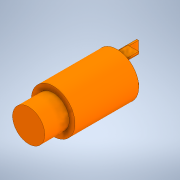
# Autodesk Inventor part: StereoBuchseEinbau
Saved by Autodesk Inventor 2020 (Build 240168000, 168)
## iProperties
Created: 2020-02-17
Part Number: StereoBuchseEinbau
Material: Generic
Document SubType Name: Modeling
Designer: Timo
Density: 1 g/cm^3
Appearance: Default
Author: Timo
Autodesk Inventor part; units mm, degrees
ref_plane "YZ Plane" through (0, 0, 0) normal (1, 0, 0) x (0, 1, 0)
ref_plane "XZ Plane" through (0, 0, 0) normal (0, 1, 0) x (-1, 0, 0)
ref_plane "XY Plane" through (0, 0, 0) normal (0, 0, 1) x (1, 0, 0)
sketch "Sketch1" plane through (0, 0, 0) normal (0, 0, 1) x (1, 0, 0)
  circle A0 centre (0, 0) radius 2.95
  dimension "d0" = 5.9
  constraints: 1 centre point, 1 coincident
  measures "d0" diameter of A0
extrude "Extrusion1" add sketch "Sketch1" along normal blind 4.5
sketch "Sketch2" plane through (0, 0, 0) normal (0, 0, -1) x (-1, 0, 0)
  circle A0 centre (0, 0) radius 4
  dimension "d3" = 8
  constraints: 1 centre point, 1 coincident
  measures "d3" diameter of A0
extrude "Extrusion2" add sketch "Sketch2" along normal blind 11.7
sketch "Sketch3" plane through (0, 0, -11.7) normal (0, 0, -1) x (-1, 0, 0)
  line L0 (2.665, 1.1) -> (2.335, 1.1)
  line L1 (2.335, 1.1) -> (2.335, -1.1)
  line L2 (2.335, -1.1) -> (2.665, -1.1)
  line L3 (2.665, -1.1) -> (2.665, 1.1)
  line L4 (2.5, 1.1) -> (2.5, -1.1) construction
  line L5 (5.6, 0) -> (-5.6, 0) construction
  point P0 (0, 0)
  point P1 (2.5, 0)
  dimension "d6" = 0.33
  dimension "d7" = 2.2
  dimension "d8" = 2.5
  constraints: 10 end point, 3 midpoint, 2 parallel, 1 horizontal, 1 perpendicular, 1 point on line
  measures "d6" distance of L1.end L2.end
  measures "d7" distance of L2.end L0.start
  measures "d8" distance from line of point (0, 0) L4
extrude "Extrusion3" add sketch "Sketch3" along normal blind 6.3
sketch "Sketch4" plane through (0, 0, -11.7) normal (0, 0, -1) x (-1, 0, 0)
  line L0 (1, 2.65) -> (-1, 2.65)
  line L1 (-1, 2.65) -> (-1, 2.35)
  line L2 (-1, 2.35) -> (1, 2.35)
  line L3 (1, 2.35) -> (1, 2.65)
  line L4 (1, -2.35) -> (-1, -2.35)
  line L5 (-1, -2.35) -> (-1, -2.65)
  line L6 (-1, -2.65) -> (1, -2.65)
  line L7 (1, -2.65) -> (1, -2.35)
  line L8 (0, -5.6) -> (0, 5.6) projected
  line L9 (1, 2.5) -> (-1, 2.5) construction
  line L10 (-1, -2.5) -> (1, -2.5) construction
  line L11 (5.6, 0) -> (-5.6, 0) construction
  point P0 (0, 0)
  point P1 (0, 2.35)
  dimension "d11" = 2
  dimension "d12" = 0.3
  dimension "d13" = 5
  constraints: 20 end point, 5 midpoint, 4 parallel, 3 collinear, 2 horizontal, 2 perpendicular, 1 point on line, 1 other
  measures "d11" distance of L0.start L0.end
  measures "d12" distance of L2.end L0.start
  measures "d13" distance between parallel lines of L10 L9
extrude "Extrusion4" add sketch "Sketch4" along normal blind 3
body "Solid1"
